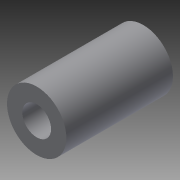
# Autodesk Inventor part: shaft coupler
Saved by Autodesk Inventor 2014 SP1 (Build 180222100, 222)
## iProperties
Created: 2014-07-17
Part Number: shaft coupler
Material: Generic
Document SubType Name: Modeling
Designer: Richard
Density: 1 g/cm^3
Appearance: Default
Author: Richard
Autodesk Inventor part; units mm, degrees
ref_plane "YZ Plane" through (0, 0, 0) normal (1, 0, 0) x (0, 1, 0)
ref_plane "XZ Plane" through (0, 0, 0) normal (0, 1, 0) x (-1, 0, 0)
ref_plane "XY Plane" through (0, 0, 0) normal (0, 0, 1) x (1, 0, 0)
sketch "Sketch1" plane through (0, 0, 0) normal (0, 0, 1) x (1, 0, 0)
  circle A0 centre (0, 0) radius 5.625
  circle A1 centre (0, 0) radius 7.375
  dimension "d0" = 11.25
  dimension "d1" = 14.75
  constraints: 2 centre point, 2 coincident
  measures "d0" diameter of A0
  measures "d1" diameter of A1
extrude "Extrusion1" add sketch "Sketch1" along normal blind 9
sketch "Sketch2" plane through (0, 0, 9) normal (0, 0, 1) x (1, 0, 0)
  circle A0 centre (0, 0) radius 7.375 projected
  circle A1 centre (0, 0) radius 7.375
  constraints: 1 centre point, 1 coincident, 1 concentric
extrude "Extrusion2" add sketch "Sketch2" along normal blind 17.5
sketch "Sketch3" plane through (0, 0, 26.5) normal (0, 0, 1) x (1, 0, 0)
  circle A0 centre (0, 0) radius 7.375 projected
  circle A1 centre (0, 0) radius 3.575
  dimension "d6" = 7.15
  constraints: 1 centre point, 1 coincident
  measures "d6" diameter of A1
extrude "Extrusion3" cut sketch "Sketch3" against normal blind 7.5 contours A1
sketch "Sketch4" plane through (0, 0, 19) normal (0, 0, 1) x (1, 0, 0)
  circle A0 centre (0, 0) radius 3.575 projected
  circle A1 centre (0, 0) radius 3.575
  constraints: 1 centre point, 1 coincident, 1 concentric
extrude "Extrusion4" cut sketch "Sketch4" against normal blind 3.2
chamfer "Chamfer1" distance 3.575 angle 45 1 edges at (-3.575, 0, 15.8)
sketch "Sketch5" plane through (0, 0, 9) normal (0, 0, -1) x (-1, 0, 0)
  circle A0 centre (0, 0) radius 5.625 projected
  line L0 (-0.6, 5.5929) -> (0, 4.125)
  line L1 (0, 4.125) -> (0.6, 5.5929)
  arc A1 (0.6, 5.5929) -> (-0.6, 5.5929) centre (0, 0) ccw
  line L2 (-3.3161, 4.5436) -> (-2.0625, 3.5724)
  line L3 (-2.0625, 3.5724) -> (-2.2768, 5.1436)
  arc A2 (-2.2768, 5.1436) -> (-3.3161, 4.5436) centre (0, 0) ccw
  line L4 (-5.1436, 2.2768) -> (-3.5724, 2.0625)
  line L5 (-3.5724, 2.0625) -> (-4.5436, 3.3161)
  arc A3 (-4.5436, 3.3161) -> (-5.1436, 2.2768) centre (0, 0) ccw
  line L6 (-5.5929, -0.6) -> (-4.125, 0)
  line L7 (-4.125, 0) -> (-5.5929, 0.6)
  arc A4 (-5.5929, 0.6) -> (-5.5929, -0.6) centre (0, 0) ccw
  line L8 (-4.5436, -3.3161) -> (-3.5724, -2.0625)
  line L9 (-3.5724, -2.0625) -> (-5.1436, -2.2768)
  arc A5 (-5.1436, -2.2768) -> (-4.5436, -3.3161) centre (0, 0) ccw
  line L10 (-2.2768, -5.1436) -> (-2.0625, -3.5724)
  line L11 (-2.0625, -3.5724) -> (-3.3161, -4.5436)
  arc A6 (-3.3161, -4.5436) -> (-2.2768, -5.1436) centre (0, 0) ccw
  line L12 (0.6, -5.5929) -> (0, -4.125)
  line L13 (0, -4.125) -> (-0.6, -5.5929)
  arc A7 (-0.6, -5.5929) -> (0.6, -5.5929) centre (0, 0) ccw
  line L14 (3.3161, -4.5436) -> (2.0625, -3.5724)
  line L15 (2.0625, -3.5724) -> (2.2768, -5.1436)
  arc A8 (2.2768, -5.1436) -> (3.3161, -4.5436) centre (0, 0) ccw
  line L16 (5.1436, -2.2768) -> (3.5724, -2.0625)
  line L17 (3.5724, -2.0625) -> (4.5436, -3.3161)
  arc A9 (4.5436, -3.3161) -> (5.1436, -2.2768) centre (0, 0) ccw
  line L18 (5.5929, 0.6) -> (4.125, 0)
  line L19 (4.125, 0) -> (5.5929, -0.6)
  arc A10 (5.5929, -0.6) -> (5.5929, 0.6) centre (0, 0) ccw
  line L20 (4.5436, 3.3161) -> (3.5724, 2.0625)
  line L21 (3.5724, 2.0625) -> (5.1436, 2.2768)
  arc A11 (5.1436, 2.2768) -> (4.5436, 3.3161) centre (0, 0) ccw
  line L22 (2.2768, 5.1436) -> (2.0625, 3.5724)
  line L23 (2.0625, 3.5724) -> (3.3161, 4.5436)
  arc A12 (3.3161, 4.5436) -> (2.2768, 5.1436) centre (0, 0) ccw
  point P0 (0, 5.625)
  point P1 (-2.8125, 4.8714)
  point P2 (-4.8714, 2.8125)
  point P3 (-5.625, 0)
  point P4 (-4.8714, -2.8125)
  point P5 (-2.8125, -4.8714)
  point P6 (0, -5.625)
  point P7 (2.8125, -4.8714)
  point P8 (4.8714, -2.8125)
  point P9 (5.625, 0)
  point P10 (4.8714, 2.8125)
  point P11 (2.8125, 4.8714)
  dimension "d16" = 1.5
  dimension "d17" = 0.6
  dimension "d18" = 0
  dimension "d19" = 0
  dimension "d20" = 0.6
  dimension "d23" = 360
  constraints: 48 end point, 39 point on circle, 12 centre point, 97 other
  measures "d16" distance of L0.end A0.start
  measures "d17" horizontal distance of A0.start L0.start
  measures "d18" horizontal distance of A0.centre A0.start
  measures "d19" horizontal distance of L0.end A0.start
  measures "d20" horizontal distance of A0.start L1.end
extrude "Extrusion5" add sketch "Sketch5" along normal blind 9 contours A0 L19 L18 | L21 L20 A0 | A0 L17 L16 | L23 L22 A0 | A0 L15 L14 | L1 L0 A0 | A0 L13 L12 | L3 L2 A0 | A0 L11 L10 | L5 L4 A0 | A0 L9 L8 | L7 L6 A0
body "Solid1"
